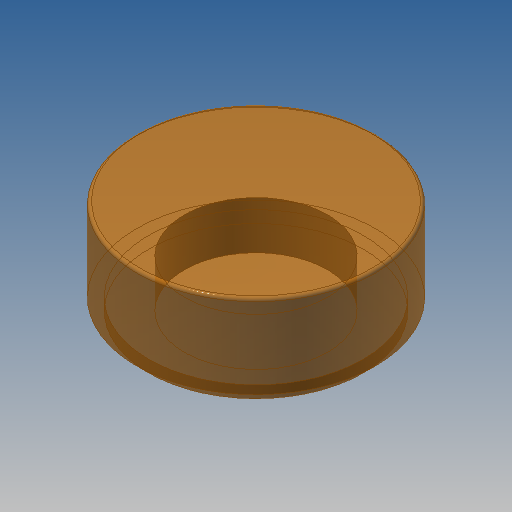
# Autodesk Inventor part: 98138-TransOrange
Saved by Autodesk Inventor 2022.2 (Build 262287000, 287)
## iProperties
Created: 2014-06-03
Part Number: 98138-TransOrange
Material: Polycarbonate
Document SubType Name: Modeling
Designer: D. Kohfeld
Density: 1.2 g/cm^3
Appearance: TransOrange
Mass: 0.153627 g
Surface Area: 2.02995 cm^2
Volume: 0.128023 cm^3
Author: D. Kohfeld
Autodesk Inventor part; units mm, degrees
ref_plane "YZ Plane" through (0, 0, 0) normal (1, 0, 0) x (0, 1, 0)
ref_plane "XZ Plane" through (0, 0, 0) normal (0, 1, 0) x (-1, 0, 0)
ref_plane "XY Plane" through (0, 0, 0) normal (0, 0, 1) x (1, 0, 0)
sketch "Sketch2" plane through (0, 0, 0) normal (0, 1, 0) x (-1, 0, 0)
  line L0 (-4, 4) -> (4, 4) construction
  line L1 (4, 4) -> (4, -4) construction
  line L2 (4, -4) -> (-4, -4) construction
  line L3 (-4, -4) -> (-4, 4) construction
  circle A0 centre (0, 0) radius 4
  point P0 (0, 4)
  point P1 (-4, 0)
  dimension "d0" = 8
  dimension "d1" = 8
  constraints: 8 end point, 2 horizontal alignment, 2 midpoint, 2 parallel, 1 coincident, 1 horizontal, 1 perpendicular, 1 vertical alignment, 2 other
  measures "d0" distance of L1.end L2.end
  measures "d1" distance of L2.end L0.start
extrude "Extrusion1" add sketch "Sketch2" along normal blind 3.2
sketch "Sketch10" plane through (0, 0, 0) normal (0, -1, 0) x (1, 0, 0)
  circle A0 centre (0, 0) radius 4 projected
  circle A1 centre (4, 4) radius 2.4 construction
  line L0 (0, 0) -> (4, 4) construction
  circle A2 centre (0, 0) radius 3.2569
  circle A3 centre (0, 0) radius 2.4
  circle A4 centre (0, 0) radius 3.6
  dimension "d92" = 4.8
  dimension "d93" = 4
  dimension "d94" = 4
  dimension "d95" = 4.8
  dimension "d99" = 0.4
  constraints: 4 centre point, 3 coincident, 2 end point, 1 tangent
  measures "d92" diameter of A1
  measures "d93" horizontal distance of L0.end L0.start
  measures "d94" horizontal distance of L0.start L0.end
  measures "d95" diameter of A3
  measures "d99" radial gap between concentric circles of A0 A4
extrude "Extrusion6" cut sketch "Sketch10" against normal blind 1.6 contours A3
extrude "Extrusion7" cut sketch "Sketch10" against normal blind 0.4 contours A0
fillet "Fillet1" radius 0.1 1 edges at (4, 3.2, 0)
equation "\"d4\" = 0.333333 * lh"
equation "\"d92\" = kd"
equation "\"d93\" = 0.5 * lu"
equation "\"d94\" = d93"
equation "\"d95\" = kd"
equation "\"d99\" = gw"
equation "\"d96\" = 0.333333 * lh - topthk"
equation "\"d100\" = gh"
equation "\"lh\" = 9.6"
equation "\"kd\" = 4.8"
equation "\"lu\" = 8"
equation "\"gw\" = 0.4"
equation "\"topthk\" = 1.6"
equation "\"gh\" = 0.4"
body "Solid1"
